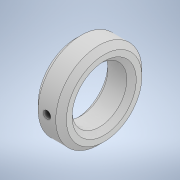
# Autodesk Inventor part: 711142
Saved by Autodesk Inventor 2022 (Build 260153000, 153)
## iProperties
Created: 2021-10-22
Part Number: 711142
Material: Типовые
Document SubType Name: Modeling
Designer: RaNSiD
Density: 1 g/cm^3
Appearance: По умолчанию
Author: RaNSiD
Autodesk Inventor part; units mm, degrees
ref_plane "YZ Plane" through (0, 0, 0) normal (1, 0, 0) x (0, 1, 0)
ref_plane "XZ Plane" through (0, 0, 0) normal (0, 1, 0) x (-1, 0, 0)
sketch "Эскиз1" plane through (-8.0178, -11.4142, 0) normal (0, 0, 1) x (1, 0, 0)
  line L0 (0, 0) -> (0, 17) construction
  line L1 (0, 20) -> (2.8284, 22.8284)
  line L2 (0, 0) -> (15, 0)
  line L3 (15, 0) -> (15, 17) construction
  line L4 (15, 20) -> (12.1716, 22.8284)
  line L5 (12.1716, 22.8284) -> (2.8284, 22.8284)
  line L6 (0, 17) -> (2.5, 14.5)
  line L7 (0, 17) -> (3.5355, 17) construction
  line L8 (2.5, 14.5) -> (12.5, 14.5)
  line L9 (12.5, 14.5) -> (15, 17)
  line L10 (12.5, 14.5) -> (16.0355, 14.5) construction
  line L11 (0, 17) -> (0, 20)
  line L12 (15, 17) -> (15, 20)
  dimension "d9" = 20
  dimension "d8" = 4
  dimension "d7" = 135
  dimension "d6" = 15
  dimension "d5" = 4
  dimension "d4" = 135
  dimension "d2" = 45
  dimension "d0" = 45
  dimension "d3" = 3
  dimension "d1" = 10
  constraints: 26 end point, 4 perpendicular, 3 equal length, 3 horizontal, 2 vertical, 1 parallel
  measures "d9" distance of L0.start L1.start
  measures "d8" distance of L1.start L1.end
  measures "d7" angle of L0 L1
  measures "d6" distance of L0.start L2.end
  measures "d5" distance of L4.start L4.end
  measures "d4" angle of L4 L3
  measures "d2" angle of L6 L7
  measures "d0" angle of L10 L9
  measures "d3" distance of L1.start L0.end
  measures "d1" distance of L6.end L8.end
revolve "Вращение1" add sketch "Эскиз1" angle 360 about axis through (-8.0178, -11.4142, 0) along (1, 0, 0)
ref_plane "РабПлоскость1" through (0, 0, 30) normal (0, 0, 1) x (1, 0, 0)
sketch "Эскиз2" plane through (0, 0, 30) normal (0, 0, 1) x (1, 0, 0)
  line L0 (-5.1893, -34.2426) -> (-5.1893, 11.4142) construction
  line L1 (4.1538, -34.2426) -> (4.1538, 11.4142) construction
  line L2 (-5.1893, 11.4142) -> (4.1538, 11.4142) construction
  point P0 (0, 0)
  point P1 (-0.5178, -11.4142)
  point P2 (-5.1893, -11.4142)
  point P3 (-0.5178, 11.4142)
  constraints: 2 midpoint, 1 horizontal alignment, 1 vertical alignment
hole "Отверстие1" at (-0.5178, -11.4142, 30) direction (0, 0, -1) diameter 4 depth 21.75
